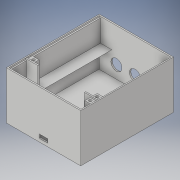
# Autodesk Inventor part: teensy_box
Saved by Autodesk Inventor 2017 (Build 210142000, 142)
## iProperties
Created: 2016-09-19
Part Number: teensy_box
Material: Generic
Document SubType Name: Modeling
Designer: corvera
Density: 1 g/cm^3
Appearance: Default
Author: corvera
Autodesk Inventor part; units mm, degrees
ref_plane "YZ Plane" through (0, 0, 0) normal (1, 0, 0) x (0, 1, 0)
ref_plane "XZ Plane" through (0, 0, 0) normal (0, 1, 0) x (-1, 0, 0)
ref_plane "XY Plane" through (0, 0, 0) normal (0, 0, 1) x (1, 0, 0)
sketch "Sketch1" plane through (0, 0, 0) normal (0, 1, 0) x (-1, 0, 0)
  line L0 (40, 50) -> (-40, 50)
  line L1 (-40, 50) -> (-40, -50)
  line L2 (-40, -50) -> (40, -50)
  line L3 (40, -50) -> (40, 50)
  line L4 (40, 50) -> (-40, -50) construction
  line L5 (-40, 50) -> (40, -50) construction
  point P0 (0, 0)
  dimension "box_width" = 80
  dimension "box_height" = 100
  constraints: 12 end point, 2 midpoint, 2 parallel, 1 horizontal, 1 perpendicular
  measures "box_width" distance of L1.end L2.end
  measures "box_height" distance of L0.end L1.end
extrude "Base" add sketch "Sketch1" against normal blind 1.5
sketch "Sketch2" plane through (0, 0, 0) normal (0, 1, 0) x (-1, 0, 0)
  line L0 (40, -50) -> (-40, -50) projected
  line L1 (40, 50) -> (-40, 50)
  line L2 (-40, 50) -> (-40, -50)
  line L3 (-40, -50) -> (40, -50)
  line L4 (40, -50) -> (40, 50)
  line L5 (40, 50) -> (-40, -50) construction
  line L6 (-40, 50) -> (40, -50) construction
  line L7 (38.8, 48.5) -> (-38.8, 48.5)
  line L8 (-38.8, 48.5) -> (-38.8, -48.5)
  line L9 (-38.8, -48.5) -> (38.8, -48.5)
  line L10 (38.8, -48.5) -> (38.8, 48.5)
  line L11 (38.8, 48.5) -> (-38.8, -48.5) construction
  line L12 (-38.8, 48.5) -> (38.8, -48.5) construction
  point P0 (0, 0)
  dimension "wall_thickness" = 1.5
  constraints: 24 end point, 4 midpoint, 4 parallel, 2 horizontal, 2 perpendicular, 1 point on line
  measures "wall_thickness" distance between parallel lines of L0 L9
extrude "Wall" add sketch "Sketch2" along normal blind 50
sketch "Sketch3" plane through (0, 0, 0) normal (0, 1, 0) x (-1, 0, 0)
  line L0 (-9.25, 49) -> (9.25, 49)
  line L1 (9.25, 49) -> (9.25, 12.2)
  line L2 (9.25, 12.2) -> (-9.25, 12.2)
  line L3 (-9.25, 12.2) -> (-9.25, 49)
  line L4 (-9.25, 49) -> (9.25, 12.2) construction
  line L5 (9.25, 49) -> (-9.25, 12.2) construction
  line L6 (0, 30.6) -> (0, 0) construction
  line L7 (10.25, 50) -> (-10.25, 50)
  line L8 (-10.25, 50) -> (-10.25, 11.2)
  line L9 (-10.25, 11.2) -> (10.25, 11.2)
  line L10 (10.25, 11.2) -> (10.25, 50)
  line L11 (10.25, 50) -> (-10.25, 11.2) construction
  line L12 (-10.25, 50) -> (10.25, 11.2) construction
  line L13 (40, 50) -> (-40, 50) projected
  point P0 (0, 50)
  dimension "d7" = 36.8
  dimension "d8" = 18.5
  dimension "d9" = 1
  dimension "d10" = 1
  constraints: 26 end point, 6 midpoint, 4 parallel, 2 horizontal, 2 perpendicular, 1 vertical
  measures "d7" distance of L0.end L1.end
  measures "d8" distance of L1.end L2.end
  measures "d9" distance between parallel lines of L2 L9
  measures "d10" distance between parallel lines of L3 L8
extrude "Teensy Wall" add sketch "Sketch3" along normal blind 10
sketch "Sketch4" plane through (40, -1.5, -50) normal (0, 0, -1) x (-1, 0, 0)
  line L0 (78.8, 51.5) -> (1.2, 51.5) construction
  line L1 (1.2, 51.5) -> (78.8, 51.5) construction
  line L2 (40, 51.5) -> (40, 15) construction
  line L3 (40, 15) -> (20, 15) construction
  circle A0 centre (20, 15) radius 6
  line L4 (40, 15) -> (40, 0) construction
  line L5 (80, 0) -> (0, 0) construction
  circle A1 centre (40, 15) radius 6
  circle A2 centre (60, 15) radius 6
  dimension "d21" = 12
  dimension "d23" = 20
  dimension "d59" = 20
  constraints: 6 end point, 3 centre point, 2 midpoint, 1 coincident, 1 horizontal, 1 perpendicular, 1 vertical, 4 other
  measures "d21" diameter of A0
  measures "d23" distance of L2.end L3.end
  measures "d59" distance of A0.centre A1.centre
extrude "BNC Holes" cut sketch "Sketch4" against normal up to surface (1.5 mm away)
sketch "Sketch7" plane through (-38.8, 0, -48.5) normal (0, 0, 1) x (1, 0, 0)
  line L0 (78.8, 50) -> (-1.2, 50) projected
  line L1 (-1.2, -1.5) -> (-1.2, 50) projected
  line L2 (-1.2, 50) -> (-1.2, 25) construction
  line L3 (-1.2, 25) -> (13.8, 25)
  line L4 (13.8, 25) -> (-1.2, 15)
  line L5 (-1.2, 15) -> (-1.2, 25)
  line L6 (38.8, 50) -> (38.8, 0) construction
  line L7 (78.8, -1.5) -> (78.8, 50)
  line L8 (78.8, 50) -> (78.8, 25) construction
  line L9 (78.8, 25) -> (63.8, 25)
  line L10 (63.8, 25) -> (78.8, 15)
  line L11 (78.8, 15) -> (78.8, 25)
  point P0 (-1.2, 30)
  dimension "d32" = 25
  dimension "d33" = 10
  dimension "d34" = 15
  constraints: 20 end point, 4 symmetric about line, 3 vertical, 1 horizontal, 1 midpoint, 1 point on line
  measures "d32" distance of L0.end L2.end
  measures "d33" distance of L4.end L2.end
  measures "d34" distance of L2.end L3.end
extrude "Battery Support" add sketch "Sketch7" along normal up to next
sketch "Sketch8" plane through (-40, -1.5, 50) normal (0, 0, 1) x (1, 0, 0)
  line L0 (78.8, 51.5) -> (1.2, 51.5) construction
  line L1 (40, 51.5) -> (40, 1.5) construction
  line L2 (35.5, 3.5) -> (44.5, 3.5)
  line L3 (44.5, 3.5) -> (44.5, 7.5)
  line L4 (44.5, 7.5) -> (35.5, 7.5)
  line L5 (35.5, 7.5) -> (35.5, 3.5)
  line L6 (35.5, 3.5) -> (44.5, 7.5) construction
  line L7 (44.5, 3.5) -> (35.5, 7.5) construction
  point P0 (40, 5.5)
  dimension "d36" = 9
  dimension "d37" = 4
  dimension "d38" = 2
  constraints: 14 end point, 3 midpoint, 2 parallel, 1 horizontal, 1 perpendicular, 1 point on line, 1 vertical
  measures "d36" distance of L2.start L2.end
  measures "d37" distance of L2.end L3.end
  measures "d38" distance from line of L2 L1.end
extrude "USB Hole" cut sketch "Sketch8" against normal up to next
sketch "Sketch9" plane through (-38.8, 25, -48.5) normal (0, 1, 0) x (1, 0, 0)
  line L0 (0, -97) -> (0, 0) projected
  line L1 (13.8, 0) -> (13.8, -97) projected
  line L2 (0, -79.5) -> (13.8, -79.5)
  line L3 (13.8, -79.5) -> (13.8, -78)
  line L4 (13.8, -78) -> (0, -78)
  line L5 (0, -78) -> (0, -79.5)
  line L6 (0, 0) -> (77.6, 0) projected
  line L7 (63.8, 0) -> (63.8, -97) projected
  line L8 (63.8, -79.5) -> (77.6, -79.5)
  line L9 (77.6, -79.5) -> (77.6, -78)
  line L10 (77.6, -78) -> (63.8, -78)
  line L11 (63.8, -78) -> (63.8, -79.5)
  line L12 (0, -97) -> (28.55, -97) projected
  line L13 (0, -79.5) -> (1.5, -79.5)
  line L14 (1.5, -79.5) -> (1.5, -97)
  line L15 (1.5, -97) -> (0, -97)
  line L16 (0, -97) -> (0, -79.5)
  line L17 (49.05, -97) -> (77.6, -97) projected
  line L18 (77.6, -79.5) -> (76.1, -79.5)
  line L19 (76.1, -79.5) -> (76.1, -97)
  line L20 (76.1, -97) -> (77.6, -97)
  line L21 (77.6, -97) -> (77.6, -79.5)
  line L22 (77.6, 0) -> (77.6, -97) projected
  line L23 (76.1, -79.5) -> (70.1, -79.5)
  line L24 (70.1, -79.5) -> (70.1, -85.5)
  line L25 (70.1, -85.5) -> (76.1, -85.5)
  line L26 (76.1, -85.5) -> (76.1, -79.5)
  line L27 (0, -78) -> (1.5, -78)
  line L28 (1.5, -78) -> (1.5, 0)
  line L29 (1.5, 0) -> (0, 0)
  line L30 (0, 0) -> (0, -78)
  line L31 (77.6, -78) -> (76.1, -78)
  line L32 (76.1, -78) -> (76.1, 0)
  line L33 (76.1, 0) -> (77.6, 0)
  line L34 (77.6, 0) -> (77.6, -78)
  line L35 (76.1, -78) -> (70.1, -78)
  line L36 (70.1, -78) -> (70.1, -72)
  line L37 (70.1, -72) -> (76.1, -72)
  line L38 (76.1, -72) -> (76.1, -78)
  line L39 (77.6, 0) -> (0, 0) projected
  line L40 (1.5, 0) -> (6.9705, 0)
  line L41 (1.5, -6.3005) -> (1.5, 0)
  line L42 (1.5, -78) -> (6.9, -78)
  line L43 (1.5, -72.6667) -> (1.5, -78)
  line L44 (1.5, -78) -> (6.9, -78)
  line L45 (1.5, -72) -> (1.5, -78)
  line L46 (1.5, -78) -> (7.5, -78)
  line L47 (7.5, -78) -> (7.5, -72)
  line L48 (7.5, -72) -> (1.5, -72)
  line L49 (1.5, -72) -> (1.5, -78)
  point P0 (38.8, -48.5)
  dimension "d41" = 78
  dimension "d42" = 1.5
  dimension "d45" = 1.5
  dimension "d47" = 1.5
  dimension "d48" = 6
  dimension "d56" = 17.5
  constraints: 84 end point, 23 equal length, 9 perpendicular, 9 point on line, 8 collinear, 6 horizontal, 1 midpoint
  measures "d41" distance between parallel lines of L6 L4
  measures "d42" distance between parallel lines of L4 L2
  measures "d45" distance between parallel lines of L16 L14
  measures "d47" distance between parallel lines of L19 L21
  measures "d48" distance of L23.end L24.end
  measures "d56" distance of L13.end L14.end
extrude "Plate Support" add sketch "Sketch9" along normal blind 23.5 contours L0 L2 L14 L12 | L0 L4 L1 L2 | L0 L6 L28 L4 | L28 L48 L47 L4 | L6 L22 L10 L32 | L10 L9 L8 L7 | L32 L10 L36 L37 | L8 L19 L25 L24 | L21 L17 L19 L8
sketch "Sketch10" plane through (-38.8, 48.5, -48.5) normal (0, 1, 0) x (1, 0, 0)
  circle A0 centre (73.1, -82.5) radius 1.45
  line L0 (63.8, -78) -> (70.1, -78) construction
  line L1 (70.1, -85.5) -> (70.1, -79.5) construction
  line L2 (70.1, -79.5) -> (73.1, -82.5) construction
  line L3 (70.1, -85.5) -> (76.1, -85.5) construction
  line L4 (73.1, -82.5) -> (76.1, -85.5) construction
  line L5 (73.1, -82.5) -> (70.1, -85.5) construction
  circle A1 centre (73.1, -75) radius 1.45
  line L6 (73.1, -75) -> (70.1, -72) construction
  line L7 (70.1, -72) -> (76.1, -72) construction
  line L8 (76.1, -72) -> (73.1, -75) construction
  line L9 (70.1, -78) -> (73.1, -75) construction
  line L10 (1.5, -72) -> (1.5, 0) projected
  line L11 (1.5, -78) -> (7.5, -78)
  line L12 (7.5, -78) -> (7.5, -72)
  line L13 (7.5, -72) -> (1.5, -72)
  line L14 (1.5, -72) -> (1.5, -78)
  line L15 (70.1, -72) -> (70.1, -78) projected
  circle A2 centre (4.5, -75) radius 1.45
  line L16 (7.5, -78) -> (7.5, -72) construction
  line L17 (4.5, -75) -> (7.5, -78) construction
  line L18 (4.5, -75) -> (7.5, -72) construction
  line L19 (4.5, -75) -> (1.5, -72) construction
  point P0 (38.8, -48.5)
  dimension "d49" = 2.9
  dimension "d52" = 2.9
  dimension "d53" = 2.9
  constraints: 26 end point, 8 equal length, 3 centre point, 2 equal radius, 2 parallel, 2 perpendicular
  measures "d49" diameter of A0
  measures "d52" diameter of A2
  measures "d53" diameter of A1
extrude "Holes" cut sketch "Sketch10" against normal blind 10 contours A0 | A1 | A2
sketch "Sketch11" plane through (-38.8, 48.5, -48.5) normal (0, 1, 0) x (1, 0, 0)
  line L0 (13.8, -79.5) -> (13.8, -78) projected
  line L1 (13.8, -78) -> (13.8, -79.5)
  line L2 (13.8, -79.5) -> (0.1333, -79.5)
  line L3 (0.1333, -79.5) -> (0.1333, -78)
  line L4 (0.1333, -78) -> (13.8, -78)
  line L5 (70.1, -78) -> (63.8, -78) projected
  line L6 (63.8, -78) -> (63.8, -79.5)
  line L7 (63.8, -79.5) -> (77.4667, -79.5)
  line L8 (77.4667, -79.5) -> (77.4667, -78)
  line L9 (77.4667, -78) -> (63.8, -78)
  point P0 (38.8, -48.5)
  constraints: 16 end point, 4 parallel, 3 perpendicular, 1 vertical
extrude "Extrusion10" add sketch "Sketch11" along normal blind 1.5
body "Solid1"
